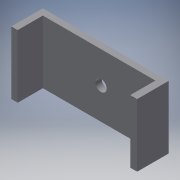
# Autodesk Inventor part: flange
Saved by Autodesk Inventor 2019 (Build 230136000, 136)
## iProperties
Created: 2021-11-02
Part Number: flange
Material: Generic
Document SubType Name: Modeling
Designer: modym
Density: 1 g/cm^3
Appearance: Default
Author: modym
Autodesk Inventor part; units mm, degrees
ref_plane "YZ Plane" through (0, 0, 0) normal (1, 0, 0) x (0, 1, 0)
ref_plane "XZ Plane" through (0, 0, 0) normal (0, 1, 0) x (-1, 0, 0)
ref_plane "XY Plane" through (0, 0, 0) normal (0, 0, 1) x (1, 0, 0)
sketch "Sketch1" plane through (0, 0, 0) normal (0, 1, 0) x (-1, 0, 0)
  line L0 (0, 0) -> (0, -20)
  line L1 (0, -20) -> (89.5, -20)
  line L2 (89.5, -20) -> (89.5, 0)
  line L3 (89.5, 0) -> (94.5, 0)
  line L4 (94.5, 0) -> (94.5, -25)
  line L5 (94.5, -25) -> (-5.5, -25)
  line L6 (-5.5, -25) -> (-5.5, 0)
  line L7 (-5.5, 0) -> (0, 0)
  line L8 (0, 1280) -> (0, -20) projected
  line L9 (89.5, -20) -> (89.5, 1280) projected
  line L10 (0, -20) -> (0, 1280) projected
  line L11 (89.5, 1280) -> (89.5, -20) projected
  dimension "d0" = 20
  dimension "d1" = 89.5
  dimension "d2" = 5
  dimension "d3" = 25
  dimension "d4" = 100
  dimension "d10" = 89.5
  dimension "d12" = 89.5
  constraints: 16 end point, 7 perpendicular, 1 point on line, 1 vertical
  measures "d0" distance of L0.start L0.end
  measures "d1" distance of L0.end L1.end
  measures "d2" distance of L2.end L3.end
  measures "d3" distance of L3.end L4.end
  measures "d4" distance of L4.end L5.end
  measures "d10" distance between parallel lines of L9 L8
  measures "d12" distance between parallel lines of L11 L10
extrude "Extrusion1" add sketch "Sketch1" along normal blind 50
sketch "Sketch2" plane through (-89.5, 0, -20) normal (0, 0, 1) x (1, 0, 0)
  line L0 (89.5, 0) -> (0, 0) projected
  line L1 (89.5, 0) -> (89.5, 50) projected
  line L2 (0, 50) -> (89.5, 50) projected
  line L3 (0, 0) -> (0, 50) projected
  circle A0 centre (46.25, 25) radius 4.5
  line L4 (-5, 0) -> (-5, 50) projected
  dimension "d7" = 9
  dimension "d11" = 51.25
  constraints: 1 centre point
  measures "d7" diameter of A0
  measures "d11" distance from line of L4 A0.centre
extrude "Extrusion2" cut sketch "Sketch2" against normal blind 50 contours A0
equation "\"d1\" = d10"
body "Solid1"
